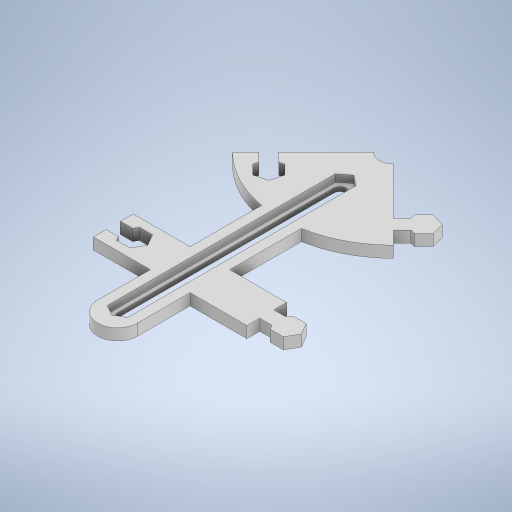
# Autodesk Inventor part: New_08_Crane_Arm_Vertical_XL
Saved by Autodesk Inventor 2024.2 (Build 282272000, 272)
## iProperties
Created: 2025-05-26
Part Number: New_08_Crane_Arm_Vertical_XL
Material: Všeobecné
Document SubType Name: Modeling
Designer: Elite
Density: 1 g/cm^3
Appearance: Výchozí
Author: Elite
Autodesk Inventor part; units mm, degrees
ref_plane "YZ Plane" through (0, 0, 0) normal (1, 0, 0) x (0, 1, 0)
ref_plane "XZ Plane" through (0, 0, 0) normal (0, 1, 0) x (-1, 0, 0)
ref_plane "XY Plane" through (0, 0, 0) normal (0, 0, 1) x (1, 0, 0)
sketch "Náčrt1" plane through (3.6, 12.9231, 50.0016) normal (0, 0, 1) x (1, 0, 0)
  line L0 (3.4, -51.2206) -> (3.4, 32.0765) projected
  line L1 (-10.6, 32.0765) -> (-10.6, -51.2206) projected
  line L2 (3.4, 32.0765) -> (-10.6, 32.0765) projected
  circle A0 centre (-3.5987, -48.8454) radius 2.0783 projected
  line L3 (0, -50.927) -> (0, 0) projected
  line L4 (-3.6, -53.0054) -> (0, -50.927) projected
  line L5 (-7.2, -50.927) -> (-3.6, -53.0054) projected
  arc A1 (-10.6, -50.9238) -> (3.4, -50.787) centre (-3.5993, -50.9238) ccw
  line L6 (3.4, -25.4635) -> (3.4, -18.4635)
  line L7 (3.4, -18.4635) -> (23.4, -18.4635)
  line L8 (23.4, -18.4635) -> (23.4, -32.4635)
  line L9 (23.4, -32.4635) -> (3.4, -32.4635)
  line L10 (3.4, -25.4635) -> (3.4, -32.4635)
  line L11 (23.4, -25.4635) -> (23.4, -22.9635)
  line L12 (23.4, -22.9635) -> (26.9, -22.9635)
  line L13 (26.9, -22.9635) -> (26.9, -27.9635)
  line L14 (26.9, -27.9635) -> (23.4, -27.9635)
  line L15 (23.4, -25.4635) -> (23.4, -27.9635)
  line L16 (35.5188, -25.4635) -> (33.2094, -29.4635)
  line L17 (33.2094, -29.4635) -> (28.5906, -29.4635)
  line L18 (28.5906, -29.4635) -> (27.7246, -27.9635)
  line L19 (27.7246, -22.9635) -> (28.5906, -21.4635)
  line L20 (28.5906, -21.4635) -> (33.2094, -21.4635)
  line L21 (33.2094, -21.4635) -> (35.5188, -25.4635)
  line L22 (26.9, -22.9635) -> (27.7246, -22.9635)
  line L23 (26.9, -27.9635) -> (27.7246, -27.9635)
  line L24 (-10.6, -25.4635) -> (-10.6, -18.4635)
  line L25 (-10.6, -18.4635) -> (-30.6, -18.4635)
  line L26 (-30.6, -18.4635) -> (-30.6, -32.4635)
  line L27 (-30.6, -32.4635) -> (-10.6, -32.4635)
  line L28 (-10.6, -25.4635) -> (-10.6, -32.4635)
  line L29 (-30.6, -25.4635) -> (-30.6, -22.9635)
  line L30 (-30.6, -25.4635) -> (-30.6, -27.9635)
  line L31 (-27.1, -27.9635) -> (-30.6, -27.9635)
  line L32 (-30.6, -22.9635) -> (-27.1, -22.9635)
  line L33 (-27.1, -22.9635) -> (-27.1, -27.9635)
  line L34 (-27.1, -22.9635) -> (-26.2754, -22.9635)
  line L35 (-27.1, -27.9635) -> (-26.2754, -27.9635)
  line L36 (-25.4094, -29.4635) -> (-26.2754, -27.9635)
  line L37 (-26.2754, -22.9635) -> (-25.4094, -21.4635)
  line L38 (-20.7906, -29.4635) -> (-25.4094, -29.4635)
  line L39 (-25.4094, -21.4635) -> (-20.7906, -21.4635)
  line L40 (-18.4812, -25.4635) -> (-20.7906, -29.4635)
  line L41 (-20.7906, -21.4635) -> (-18.4812, -25.4635)
  line L42 (-3.6, 32.0765) -> (-3.6, 46.0765)
  arc A2 (-31.8843, 17.7922) -> (24.6843, 17.7922) centre (-3.6, 46.0765) ccw
  line L43 (-3.6, 46.0765) -> (-31.8843, 17.7922)
  line L44 (-3.6, 46.0765) -> (24.6843, 17.7922)
  line L45 (-3.6, 46.0765) -> (48.0562, 46.0765) construction
  line L46 (-25.5203, 24.1562) -> (-23.7525, 25.9239)
  line L47 (-25.5203, 24.1562) -> (-27.2881, 22.3884)
  line L48 (-24.8132, 19.9135) -> (-27.2881, 22.3884)
  line L49 (-23.7525, 25.9239) -> (-21.2777, 23.4491)
  line L50 (-21.2777, 23.4491) -> (-24.8132, 19.9135)
  line L51 (-21.2777, 23.4491) -> (-20.6946, 22.866)
  line L52 (-24.8132, 19.9135) -> (-24.2301, 19.3305)
  line L53 (-20.6946, 22.866) -> (-19.0216, 23.3143)
  line L54 (-24.6784, 17.6574) -> (-24.2301, 19.3305)
  line L55 (-19.0216, 23.3143) -> (-15.7556, 20.0483)
  line L56 (-16.951, 15.5869) -> (-21.4124, 14.3914)
  line L57 (-15.7556, 20.0483) -> (-16.951, 15.5869)
  line L58 (-21.4124, 14.3914) -> (-24.6784, 17.6574)
  line L59 (26.8896, 32.7254) -> (28.085, 28.264)
  line L60 (22.4282, 33.9209) -> (26.8896, 32.7254)
  line L61 (28.085, 28.264) -> (24.819, 24.998)
  line L62 (19.1622, 30.6549) -> (22.4282, 33.9209)
  line L63 (18.3203, 24.1562) -> (16.5525, 25.9239)
  line L64 (19.6105, 28.9819) -> (19.1622, 30.6549)
  line L65 (24.819, 24.998) -> (23.146, 25.4463)
  line L66 (19.0274, 28.3988) -> (19.6105, 28.9819)
  line L67 (19.0274, 28.3988) -> (22.563, 24.8633)
  line L68 (22.563, 24.8633) -> (23.146, 25.4463)
  line L69 (22.563, 24.8633) -> (20.0881, 22.3884)
  line L70 (18.3203, 24.1562) -> (20.0881, 22.3884)
  line L71 (16.5525, 25.9239) -> (19.0274, 28.3988)
  line L72 (24.6843, 17.7922) -> (18.3203, 24.1562)
  circle A3 centre (-3.6, 46.0765) radius 5
  line L73 (-7.2, -50.927) -> (-7.2, 32.0765)
  line L74 (0, -50.927) -> (0, 32.0765)
  line L75 (-7.2, 29.2565) -> (-3.6, 32.0765)
  line L76 (-3.6, 32.0765) -> (0, 29.2565)
  line L77 (-3.6, 29.2565) -> (-1.5215, 29.2565) construction
  circle A4 centre (-3.6, 27.178) radius 2.0785
  line L78 (-5.6785, 27.1779) -> (-5.677, -48.8455)
  line L79 (-1.5215, 27.1779) -> (-1.5203, -48.8454)
  point P0 (30.9, -25.4635)
  point P1 (26.9, -25.4635)
  point P2 (-27.1, -25.4635)
  point P3 (-23.1, -25.4635)
  point P4 (-23.0454, 21.6813)
  point P5 (-20.217, 18.8529)
  point P6 (23.4958, 25.7125)
  point P7 (23.6236, 29.4595)
  point P8 (20.7952, 26.631)
  point P9 (-10.6, 6.6937)
  point P10 (3.4, 6.6937)
  point P11 (16.5525, 25.9239)
  point P12 (-0.0645, 42.5409)
  point P13 (-7.1355, 42.5409)
  dimension "d4" = 7
  dimension "d5" = 20
  dimension "k" = 14
  dimension "d9" = 3.5
  dimension "d10" = 5
  dimension "d14" = 8
  dimension "d15" = 4
  dimension "d16" = 7
  dimension "d19" = 14
  dimension "d21" = 45
  dimension "d22" = 40
  dimension "d24" = 10
  dimension "d34" = 4.1567
  dimension "d35" = 2.0817
  dimension "d36" = 2.82
  constraints: 148 end point, 14 point on line, 10 point on circle, 6 perpendicular, 5 horizontal, 4 centre point, 4 tangent, 3 midpoint, 2 coincident, 2 collinear, 1 parallel, 1 vertical, 11 other
  measures "d4" distance of L6.start L6.end
  measures "d5" distance of L6.end L7.end
  measures "k" distance of L7.end L8.end
  measures "d9" distance of L11.end L12.end
  measures "d10" distance of L12.end L13.end
  measures "d14" distance between parallel lines of L17 L20
  measures "d15" distance of point (26.9, -25.463) point (30.9, -25.463)
  measures "d16" distance from line of L7 point (26.9, -25.463)
  measures "d19" distance of L42.start L42.end
  measures "d21" angle of L44 L45
  measures "d22" radius of A2
  measures "d24" diameter of A3
  measures "d34" diameter of A0
  measures "d35" distance of L4.start A0.start
  measures "d36" distance of L42.start L77.start
extrude "Vysunutí1" add sketch "Náčrt1" against normal blind 4 contours A1 L1 A2 L73 L5 L4 L3 L74 L0 | A2 L74 L2 L0 | L74 L3 L4 L5 L73 A2 L78 A0 L79 | A2 L79 A4 L78 L73 L75 L76 L74 | L1 L2 L73 A2 | L74 L76 L2 | L79 A0 L78 A2 | A2 L78 A4 L79 | L75 L73 L2 | A4 | A0
extrude "Vysunutí2" cut sketch "Náčrt1" against normal blind 2.5 contours L74 L3 L4 L5 L73 A2 L78 A0 L79 | A2 L79 A4 L78 L73 L75 L76 L74 | L79 A0 L78 A2 | A2 L78 A4 L79 | A4 | A0
extrude "Vysunutí3" add sketch "Náčrt1" against normal blind 4 contours L0 L7 L8 L9 | L27 L26 L31 L35 L36 L38 L40 L41 L39 L37 L34 L32 L25 L1 | L8 L12 L13 L14 | L13 L22 L19 L20 L21 L16 L17 L18 L23
extrude "Vysunutí4" add sketch "Náčrt1" against normal blind 4 contours L0 L2 L42 A3 L44 A2 | A2 L43 L48 L52 L54 L58 L56 L57 L55 L53 L51 L49 A3 L42 L2 L1 | L44 L71 L67 L69 | L67 L66 L64 L62 L60 L59 L61 L65 L68
sketch "Náčrt2" plane through (3.6, 12.9231, 50.0016) normal (0, 0, 1) x (1, 0, 0)
  line L0 (-7.2, 0) -> (-3.6, 2.0785) projected
  line L1 (-3.6, 2.0785) -> (0, 0) projected
  arc A0 (-1.525, -2.1008) -> (-5.675, -2.1796) centre (-3.6012, -2.0791) ccw projected
  line L2 (-5.675, -2.1796) -> (-5.675, -48.7542) projected
  line L3 (-1.525, -48.7062) -> (-1.525, -2.1008) projected
  arc A1 (-5.675, -48.7542) -> (-1.525, -48.7062) centre (-3.5987, -48.8454) ccw projected
  line L4 (-3.6, -53.0054) -> (-7.2, -50.927) projected
  line L5 (-7.2, -50.927) -> (-7.2, 0) projected
  line L6 (0, -50.927) -> (-3.6, -53.0054) projected
  line L7 (0, 29.2565) -> (0, -50.927) projected
  line L8 (-7.2, 35) -> (-3.6, 37.0785)
  line L9 (-3.6, 37.0785) -> (0, 35)
  line L10 (-7.2, 0) -> (-7.2, 35)
  line L11 (0, 0) -> (0, 35)
  circle A2 centre (-3.6012, -2.0791) radius 2.0763
  circle A3 centre (-3.601, 32.9202) radius 2.0763
  line L12 (-3.6406, -0.0032) -> (-3.6, 2.0785)
  line L13 (-5.675, -2.1796) -> (-5.6773, 32.9201)
  line L14 (-1.525, -2.1008) -> (-1.5247, 32.9202)
  line L15 (-7.2, 0) -> (-5.6752, 0.8803)
  line L16 (-5.6752, 0.8803) -> (-3.6, 2.0785)
  line L17 (-3.6, 2.0785) -> (-1.525, 0.8804)
  line L18 (-1.525, 0.8804) -> (0, 0)
  point P0 (-3.6, -12.9231)
  dimension "d27" = 35
  dimension "d28" = 37.0817
  dimension "d" = 4.1525
  dimension "d30" = 4.1525
  dimension "d31" = 4.1583
  dimension "d32" = 3.6012
  dimension "d33" = 3.601
  constraints: 22 end point, 4 point on line, 3 point on circle, 2 centre point, 2 collinear, 2 parallel, 2 tangent, 1 coincident, 1 vertical
  measures "d27" distance of L0.end L8.end
  measures "d28" distance of L8.end L12.start
  measures "d" diameter of A2
  measures "d30" diameter of A3
  measures "d31" distance of L8.end A3.centre
  measures "d32" distance from line of L7 A0.centre
  measures "d33" distance from line of L11 A3.centre
extrude "Vysunutí5" cut sketch "Náčrt1" against normal through all contours L79 A0 L78 A2 | A2 L78 A4 L79 | A4 | A0
equation "\"d16\" = 0.5 * k"
equation "\"d30\" = d"
